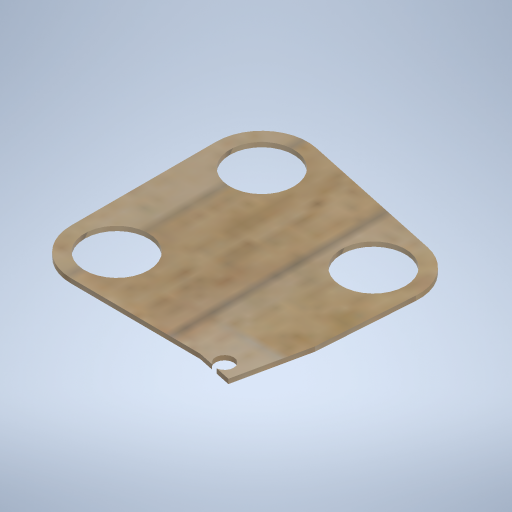
# Autodesk Inventor part: gear_plate_base
Saved by Autodesk Inventor 2024.1 (Build 281209000, 209)
## iProperties
Created: 2024-04-01
Part Number: gear_plate_base
Material: 木材 (カエデ材)
Document SubType Name: Modeling
Designer: hibik
Density: 0.67 g/cm^3
Appearance: ナチュラル カエデ材 - 光沢 濃い着色
Author: hibik
Autodesk Inventor part; units mm, degrees
ref_plane "YZ Plane" through (0, 0, 0) normal (1, 0, 0) x (0, 1, 0)
ref_plane "XZ Plane" through (0, 0, 0) normal (0, 1, 0) x (-1, 0, 0)
ref_plane "XY Plane" through (0, 0, 0) normal (0, 0, 1) x (1, 0, 0)
sketch "スケッチ1" plane through (0, 0, 0) normal (0, 1, 0) x (-1, 0, 0)
  line L0 (25, 0) -> (-25, 0)
  line L1 (-25, 0) -> (-25, -104.5)
  line L2 (-25, -104.5) -> (25, -104.5) construction
  line L3 (25, -104.5) -> (25, 0)
  circle A0 centre (0, 0) radius 25
  circle A1 centre (0, 0) radius 57 construction
  circle A2 centre (0, -79.5) radius 22.5 construction
  circle A3 centre (0, 0) radius 75 construction
  circle A4 centre (0, -79.5) radius 10.75
  circle A5 centre (0, 0) radius 10.75
  circle A6 centre (-77.7461, -62.8931) radius 25
  circle A7 centre (-77.7461, -62.8931) radius 10.75
  circle A8 centre (0, -79.5) radius 25
  line L4 (-5.2223, -103.9485) -> (-82.9684, -87.3415)
  line L5 (-72.5238, -38.4446) -> (5.2223, -55.0515)
  line L6 (-77.7461, -62.8931) -> (-82.9684, -87.3415)
  point P0 (25, -79.5)
  point P1 (-25, -48.5959)
  dimension "d0" = 114
  dimension "d1" = 45
  dimension "d2" = 150
  dimension "d4" = 21.5
  dimension "d5" = 50
  dimension "d25" = 79.5
  constraints: 14 end point, 9 centre point, 9 tangent, 8 coincident, 5 point on circle, 3 equal radius, 2 parallel, 2 perpendicular, 1 horizontal, 1 midpoint, 1 vertical alignment
  measures "d0" diameter of A1
  measures "d1" diameter of A2
  measures "d2" diameter of A3
  measures "d4" diameter of A5
  measures "d5" distance of L1.end L2.end
  measures "d25" distance from line of A2.centre L6
extrude "押し出し1" add sketch "スケッチ1" along normal blind 2.5 contours A0 L0 A5 | L0 A5 A0 | L3 A8 L5 L1 A0 | A8 | A8 L1 L5 | L4 L1 A8 | L1 L4 A6 L5 | A6
sketch "スケッチ4" plane through (0, 2.5, 0) normal (0, 1, 0) x (1, 0, 0)
  line L0 (-1, 90.2034) -> (1, 90.2034)
  line L1 (1, 90.2034) -> (1, 96.5)
  line L2 (1, 96.5) -> (-1, 96.5)
  line L3 (-1, 96.5) -> (-1, 90.2034)
  arc A0 (-25, 0) -> (25, 0) centre (0, 0) ccw projected
  line L4 (25, 0) -> (25, 48.5959) projected
  line L5 (25, 48.5959) -> (72.5238, 38.4446) projected
  arc A1 (72.5238, 38.4446) -> (82.9684, 87.3415) centre (77.7461, 62.8931) ccw projected
  line L6 (82.9684, 87.3415) -> (5.2223, 103.9485) projected
  arc A2 (5.2223, 103.9485) -> (-25, 79.5) centre (0, 79.5) ccw projected
  line L7 (-25, 79.5) -> (-25, 0) projected
  circle A3 centre (0, 0) radius 10.75 projected
  circle A4 centre (77.7461, 62.8931) radius 10.75 projected
  circle A5 centre (0, 79.5) radius 10.75 projected
  circle A6 centre (0, 79.5) radius 10.75 projected
  line L8 (-16.9706, -1) -> (16.9706, -1)
  line L9 (16.9706, -1) -> (16.9706, 1)
  line L10 (16.9706, 1) -> (-16.9706, 1)
  line L11 (-16.9706, 1) -> (-16.9706, -1)
  line L12 (-1, -16.9706) -> (1, -16.9706)
  line L13 (1, -16.9706) -> (1, 16.9706)
  line L14 (1, 16.9706) -> (-1, 16.9706)
  line L15 (-1, 16.9706) -> (-1, -16.9706)
  circle A7 centre (0, 0) radius 17
  point P0 (0, 96.5)
  point P1 (-16.9706, 0)
  point P2 (0, 16.9706)
  point P3 (-1, -10.7034)
  point P4 (1, -10.7034)
  point P5 (10.7034, 1)
  point P6 (10.7034, -1)
  point P7 (-1, 10.7034)
  point P8 (1, 10.7034)
  point P9 (-10.7034, -1)
  point P10 (-10.7034, 1)
  dimension "d26" = 17
  dimension "d27" = 2
  dimension "d30" = 34
  constraints: 24 end point, 6 parallel, 5 perpendicular, 4 point on circle, 3 horizontal, 3 midpoint, 2 vertical alignment, 1 centre point, 1 coincident, 1 horizontal alignment, 2 other
  measures "d26" distance from line of L2 A2.centre
  measures "d27" distance of L1.end L2.end
  measures "d30" diameter of A7
extrude "押し出し4" cut sketch "スケッチ4" against normal through all contours A5 L0 | L3 L2 L1 A5 | A3 L10 L9 L8 | A3 L15 L14 L13 | L13 L12 L15 A3 | A3 L8 L11 L10 picked at (-0.1113, 90.2172)
sketch "スケッチ5" plane through (0, 2.5, 0) normal (0, 1, 0) x (1, 0, 0)
  circle A0 centre (0, 0) radius 17.5
  circle A1 centre (0, 79.5) radius 17.5
  circle A2 centre (77.7461, 62.8931) radius 17.5
  arc A3 (-1, 90.2034) -> (1, 90.2034) centre (0, 79.5) ccw projected
  circle A4 centre (77.7461, 62.8931) radius 10.75 projected
  dimension "d31" = 35
  dimension "d32" = 35
  dimension "d33" = 35
  constraints: 3 centre point, 2 concentric, 1 coincident
  measures "d31" diameter of A0
  measures "d32" diameter of A1
  measures "d33" diameter of A2
extrude "押し出し5" cut sketch "スケッチ5" against normal through all contours A0 | A1 | A2 | A4
sketch "スケッチ7" plane through (0, 2.5, 0) normal (0, 1, 0) x (1, 0, 0)
  line L0 (62.2228, 90.7503) -> (63.2008, 90.5415) projected
  line L1 (62.7118, 90.6459) -> (67.0985, 111.1826)
  line L2 (9.4001, 123.5072) -> (87.1463, 106.9003) projected
  circle A0 centre (50.445, 105.0256) radius 1.75
  circle A1 centre (21.1068, 111.2923) radius 1.75
  point P0 (0, 0)
  dimension "d39" = 9.5
  dimension "d40" = 3.5
  dimension "d41" = 15
  dimension "d42" = 45
  dimension "d43" = 9.5
  constraints: 2 centre point, 2 end point, 1 equal radius, 1 midpoint, 1 perpendicular, 1 point on line
  measures "d39" distance from line of A0.centre L2
  measures "d40" diameter of A0
  measures "d41" distance from line of L1 A0.centre
  measures "d42" distance from line of A1.centre L1
  measures "d43" distance from line of L2 A1.centre
extrude "押し出し7" cut sketch "スケッチ7" against normal through all
sketch "スケッチ8" plane through (0, 2.5, 0) normal (0, 1, 0) x (1, 0, 0)
  line L0 (15.7233, -19.4365) -> (93.4694, 43.4566)
  arc A0 (-25, 0) -> (25, 0) centre (0, 0) ccw projected
  arc A1 (72.5238, 38.4446) -> (82.9684, 87.3415) centre (77.7461, 62.8931) ccw projected
  line L1 (25, 0) -> (25, 42.4151) projected
  line L2 (25, 0) -> (25, 48.5959) projected
  line L3 (25, 48.5959) -> (72.5238, 38.4446) projected
  constraints: 2 end point, 2 point on circle, 2 tangent
extrude "押し出し8" add sketch "スケッチ8" against normal up to surface (2.5 mm away)
sketch "スケッチ9" plane through (0, 2.5, 0) normal (0, 1, 0) x (1, 0, 0)
  circle A0 centre (0, 0) radius 17.5 projected
  circle A1 centre (0, 0) radius 70 construction
  circle A2 centre (0, 0) radius 75 construction
  line L0 (-14.6224, -68.4557) -> (92.9508, -91.4338)
  line L1 (82.9684, 87.3415) -> (5.2223, 103.9485) projected
  line L2 (0, 0) -> (-14.6224, -68.4557)
  line L3 (58.723, -84.1226) -> (78.2817, -88.3005)
  line L4 (78.2817, -88.3005) -> (90.8153, -29.6241)
  line L5 (90.8153, -29.6241) -> (71.2565, -25.4463)
  line L6 (71.2565, -25.4463) -> (58.723, -84.1226)
  line L7 (71.2565, -25.4463) -> (90.8153, -29.6241)
  line L8 (90.8153, -29.6241) -> (99.1709, 9.4934)
  line L9 (99.1709, 9.4934) -> (79.6122, 13.6713)
  line L10 (79.6122, 13.6713) -> (71.2565, -25.4463)
  line L11 (93.4694, 43.4566) -> (15.7233, -19.4365) projected
  arc A3 (93.4694, 43.4566) -> (82.9684, 87.3415) centre (77.7461, 62.8931) ccw projected
  line L12 (99.1709, 9.4934) -> (102.6885, 61.1962)
  line L13 (71.2565, -25.4463) -> (-0.1564, -24.9995)
  arc A4 (-25, 0) -> (15.7233, -19.4365) centre (0, 0) ccw projected
  point P0 (90.8153, -29.6241)
  dimension "d48" = 140
  dimension "d49" = 5
  dimension "d50" = 110
  dimension "d51" = 60
  dimension "d52" = 15
  dimension "d53" = 20
  dimension "d54" = 40
  constraints: 24 end point, 5 parallel, 3 perpendicular, 2 coincident, 2 collinear, 2 point on circle, 2 point on line, 2 tangent, 1 centre point, 4 other
  measures "d50" distance from line of L0.end L2
  measures "d51" distance between parallel lines of L0 L5
  measures "d52" distance from line of L4 L0.end
  measures "d53" distance between parallel lines of L6 L4
  measures "d54" distance between parallel lines of L5 L9
extrude "押し出し9" add sketch "スケッチ9" against normal up to surface (2.5 mm away) contours L10 L9 L8 L5 | L13 A4 L11 A3 L12 L9 L10
sketch "スケッチ10" plane through (0, 0, 0) normal (0, -1, 0) x (1, 0, 0)
  circle A0 centre (82.0177, 22.9389) radius 1.6 projected
  circle A1 centre (82.0177, 22.9389) radius 5
  point P0 (0, 0)
  dimension "d57" = 10
  constraints: 1 centre point, 1 coincident
  measures "d57" diameter of A1
extrude "押し出し10" cut sketch "スケッチ10" against normal through all contours A0 | A1
equation "\"d43\" = d39"
